008 (Autodesk Fusion 360 design; units mm, degrees)
Autodesk Fusion 360 part; units mm, degrees
sketch "Esquisse1" plane through (0, 0, 0) normal (0, 0, 1) x (1, 0, 0)
  line L0 (-57.5, 20) -> (57.5, 20)
  line L1 (57.5, 20) -> (57.5, -20)
  line L2 (57.5, -20) -> (-57.5, -20)
  line L3 (-57.5, -20) -> (-57.5, 20)
  line L4 (0, 1.75) -> (0, 22.5)
  line L5 (1.75, 0) -> (22.5, 0)
  dimension "d1" = 115
  dimension "d2" = 40
  constraint horizontal L0
  constraint vertical L1
  constraint horizontal L2
  constraint vertical L3
  constraint symmetric L1 L3 L4
  constraint symmetric L0 L2 L5
  measures "d1" distance of L0.start L0.end
  measures "d2" distance of L0.start L2.end
extrude "Extrusion1" add sketch "Esquisse1" along normal blind 30
sketch "Esquisse2" plane through (0, 0, 30) normal (0, 0, 1) x (-1, 0, 0)
  line L0 (57.5, 20) -> (-57.5, 20)
  line L1 (-57.5, 20) -> (-57.5, -20)
  line L2 (-57.5, -20) -> (57.5, -20)
  line L3 (57.5, -20) -> (57.5, 20)
  circle A0 centre (40, 0) radius 7.625
  line L4 (0, -1.75) -> (0, -22.5)
  line L5 (-1.75, 0) -> (-22.5, 0)
  dimension "d5" = 15.25
  dimension "d6" = 40
  constraint coincident A0.centre L5
  measures "d5" diameter of A0
  measures "d6" distance of A0.centre L4
extrude "Extrusion2" cut sketch "Esquisse2" against normal blind 25 contours A0
mirror "Symétrie miroir1" about plane through (0, 0, 0) normal (1, 0, 0) of "Extrusion2"
sketch "Esquisse3" plane through (0, 0, 30) normal (0, 0, 1) x (-1, 0, 0)
  circle A0 centre (-40, 0) radius 7.625
  circle A1 centre (40, 0) radius 7.625
  line L0 (57.5, 20) -> (-57.5, 20)
  line L1 (-57.5, 20) -> (-57.5, -20)
  line L2 (-57.5, -20) -> (57.5, -20)
  line L3 (57.5, -20) -> (57.5, 20)
sketch "Esquisse4" plane through (0, 0, 30) normal (0, 0, 1) x (1, 0, 0)
  circle A0 centre (-40, 0) radius 12 construction
  line L0 (1.75, 0) -> (22.5, 0)
  point P0 (-52, 0)
  dimension "d11" = 24
  dimension "d12" = 40
  constraint coincident A0 P0
  constraint coincident P0 L0
  constraint coincident A0.centre L0
  measures "d11" diameter of A0
  measures "d12" horizontal distance of origin A0.centre
sketch "Esquisse5" plane through (0, 0, 30) normal (0, 0, 1) x (1, 0, 0)
  circle A0 centre (0, 0) radius 5.15
  dimension "d20" = 10.3
  constraint coincident A0.centre origin
  measures "d20" diameter of A0
extrude "Extrusion3" cut sketch "Esquisse5" against normal blind 75
sketch "Esquisse6" plane through (0, 0, 30) normal (0, 0, 1) x (1, 0, 0)
  point P0 (-8, 0)
  dimension "d23" = 8
  measures "d23" distance of P0 origin
hole "Perçage2" at (-8, 0, 30) direction (0, 0, -1) diameter 4.5 depth 50 tip angle 118
pattern_circular "Réseau C2" count 4 over 360 about axis through (0, 0, 30) along (0, 0, -1) of "Perçage2"
sketch "Esquisse7" plane through (0, 0, 30) normal (0, 0, 1) x (1, 0, 0)
sketch "Esquisse8" plane through (0, 0, 30) normal (0, 0, 1) x (-1, 0, 0)
  circle A0 centre (40, 0) radius 5
  dimension "d31" = 10
  measures "d31" diameter of A0
extrude "Extrusion4" cut sketch "Esquisse8" against normal blind 51
mirror "Symétrie miroir4" about plane through (0, 0, 0) normal (1, 0, 0) of "Extrusion4"
sketch "Esquisse9" plane through (0, 0, 0) normal (0, 0, 1) x (1, 0, 0)
  circle A0 centre (-40, 0) radius 10
  dimension "d36" = 20
  measures "d36" diameter of A0
extrude "Extrusion5" add sketch "Esquisse9" against normal blind 25
sketch "Esquisse10" plane through (0, 0, -25) normal (0, 0, -1) x (1, 0, 0)
  circle A0 centre (-40, 0) radius 10
sketch "Esquisse11" plane through (0, 0, -25) normal (0, 0, -1) x (1, 0, 0)
  circle A0 centre (-40, 0) radius 7.625
  dimension "d39" = 15.25
  measures "d39" diameter of A0
extrude "Extrusion6" cut sketch "Esquisse11" against normal blind 25
mirror "Symétrie miroir5" about plane through (0, 0, 0) normal (1, 0, 0) of "Extrusion5", "Extrusion6"
sketch "Esquisse12" plane through (0, 20, 0) normal (0, 1, 0) x (-1, 0, 0)
  line L0 (-57.5, 0) -> (57.5, 0)
  line L1 (57.5, 0) -> (57.5, 30)
  line L2 (57.5, 30) -> (-57.5, 30)
  line L3 (-57.5, 30) -> (-57.5, 0)
  circle A0 centre (0, 15) radius 6
  dimension "d44" = 12
  measures "d44" diameter of A0
extrude "Extrusion7" cut sketch "Esquisse12" against normal blind 4 contours A0
sketch "Esquisse13" plane through (0, 20, 0) normal (0, 1, 0) x (-1, 0, 0)
  circle A0 centre (0, 15) radius 6
  line L0 (-57.5, 0) -> (57.5, 0)
  line L1 (57.5, 0) -> (57.5, 30)
  line L2 (57.5, 30) -> (-57.5, 30)
  line L3 (-57.5, 30) -> (-57.5, 0)
sketch "Esquisse14" plane through (0, 20, 0) normal (0, 1, 0) x (-1, 0, 0)
  line L0 (57.5, 0) -> (-57.5, 0)
  point P0 (12, 15)
  point P1 (0, 15)
  dimension "d47" = 12
  dimension "d48" = 15
  measures "d47" distance of P0 P1
  measures "d48" distance of P0 L0
hole "Perçage3" at (-12, 20, 15) direction (0, -1, 0) diameter 2.6 depth 16 tip angle 118
mirror "Symétrie miroir6" about plane through (0, 0, 0) normal (1, 0, 0) of "Perçage3"
sketch "Esquisse15" plane through (-57.5, 0, 0) normal (-1, 0, 0) x (0, -1, 0)
  line L0 (-20, 0) -> (20, 0)
  line L1 (20, 0) -> (20, 30)
  line L2 (20, 30) -> (-20, 30)
  line L3 (-20, 30) -> (-20, 0)
  circle A0 centre (0, 15) radius 6
  line L4 (20, 0) -> (-20, 0)
  dimension "d54" = 12
  dimension "d55" = 15
  dimension "d56" = 20
  measures "d54" diameter of A0
  measures "d55" distance of A0.centre L4
  measures "d56" distance of L1 A0.centre
extrude "Extrusion8" cut sketch "Esquisse15" against normal blind 5 contours A0
sketch "Esquisse16" plane through (-57.5, 0, 0) normal (-1, 0, 0) x (0, -1, 0)
  circle A0 centre (0, 15) radius 6
  line L0 (-20, 0) -> (20, 0)
  line L1 (20, 0) -> (20, 30)
  line L2 (20, 30) -> (-20, 30)
  line L3 (-20, 30) -> (-20, 0)
  line L4 (20, 0) -> (-20, 0)
  point P0 (12, 15)
  dimension "d59" = 12
  dimension "d60" = 15
  measures "d59" distance of A0.centre P0
  measures "d60" distance of P0 L4
hole "Perçage4" at (-57.5, -12, 15) direction (1, 0, 0) diameter 2.6 depth 16 tip angle 118
mirror "Symétrie miroir7" about plane through (0, 0, 0) normal (0, 1, 0) of "Perçage4"
mirror "Symétrie miroir8" about plane through (0, 0, 0) normal (1, 0, 0) of "Extrusion8", "Perçage4", "Symétrie miroir7"
equation "d23 = ( 19.5 / 2 ) * 1 mm - ( 3.5 / 2 ) * 1 mm"
